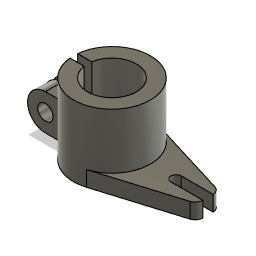
7.2 Project surface tools (Autodesk Fusion 360 design; units mm, degrees)
Autodesk Fusion 360 part; units mm, degrees
note: some values were not read from the file. Chosen so that the rebuilt part matches the saved one: which bodies a step acts on.
sketch "Sketch1" plane through (0, 0, 0) normal (0, 1, 0) x (1, 0, 0)
  circle A0 centre (0, 0) radius 19
  circle A1 centre (0, 0) radius 30
  line L0 (0, 0) -> (50, 0) construction
  line L1 (50, 0) -> (75, 0) construction
  line L2 (50, 4) -> (75, 4)
  line L3 (50, -4) -> (75, -4)
  line L4 (8.7717, 28.689) -> (70.7543, 9.7378)
  arc A2 (75, 4) -> (70.7543, 9.7378) centre (69, 4) ccw
  arc A3 (50, 4) -> (50, -4) centre (50, 0) ccw
  line L5 (8.7717, -28.689) -> (70.7543, -9.7378)
  arc A4 (70.7543, -9.7378) -> (75, -4) centre (69, -4) ccw
  dimension "d1" = 38
  dimension "d2" = 60
  dimension "d3" = 50
  dimension "d4" = 8
  dimension "d5" = 25
  dimension "d6" = 4
  dimension "d7" = 4
  dimension "d8" = 12
  constraint coincident A0.centre A1.centre
  constraint horizontal L0
  constraint coincident L0.end L1.start
  constraint parallel L0 L1
  constraint tangent A1 L4
  constraint coincident L2 A2.centre
  constraint tangent L4 A2
  constraint coincident A1 L4.start
  constraint symmetric L0 L2.end L3.end
  constraint symmetric L0 L4.end L5.end
  constraint symmetric L0 A2 A4
  constraint symmetric L0 L4.start L5.start
  measures "d1" diameter of A0
  measures "d2" diameter of A1
  measures "d3" distance of A0.centre L0.end
  measures "d4" diameter of A3
  measures "d5" distance of L0.end L1.end
  measures "d8" diameter of A2
extrude "Extrude1" add sketch "Sketch1" along normal blind 44 contours A1 makes body 1
extrude "Extrude2" add sketch "Sketch1" along normal blind 12 contours A1 L2 L3 L4 A2 A3 L5 A4 bodies 1
sketch "Sketch2" plane through (0, 0, 0) normal (0, 0, 1) x (1, 0, 0)
  circle A0 centre (-36, 22) radius 6
  line L0 (-36, 36) -> (-22, 36)
  line L1 (-22, 36) -> (-22, 8)
  line L2 (-22, 8) -> (-36, 8)
  arc A1 (-36, 36) -> (-36, 8) centre (-36, 22) ccw
  line L3 (30, 0) -> (-30, 0)
  dimension "d14" = 28
  dimension "d15" = 12
  dimension "d16" = 8
  dimension "d17" = 36
  constraint concentric A0 A1
  constraint horizontal L0
  constraint vertical L1
  constraint horizontal L2
  constraint tangent L2 A1
  constraint tangent L1 A1
  measures "d14" diameter of A1
  measures "d15" diameter of A0
  measures "d16" distance of L2 L3
  measures "d17" horizontal distance of origin A0.centre
extrude "Extrude3" add sketch "Sketch2" along normal mid plane 32 bodies 1
sketch "Sketch3" plane through (0, 44, 0) normal (0, 1, 0) x (-1, 0, 0)
  circle A0 centre (0, 0) radius 19
  circle A1 centre (0, 0) radius 30
  line L0 (54, -3) -> (11, -3)
  line L1 (11, -3) -> (11, 3)
  line L2 (11, 3) -> (54, 3)
  line L3 (54, 3) -> (54, -3)
  line L4 (0, 0) -> (-50, 0)
  dimension "d20" = 3
  dimension "d21" = 3
  dimension "d22" = 11
  dimension "d23" = 43
  constraint horizontal L0
  constraint vertical L1
  constraint horizontal L2
  constraint vertical L3
  measures "d20" distance of L0 L4
  measures "d21" distance of L2 L4
  measures "d22" distance of A0.centre L1
  measures "d23" distance of L1 L3
extrude "Extrude4" cut sketch "Sketch3" against normal up to surface (44 mm away) contours A0 A1 L0 L2 | A1 L0 L2 L3 bodies 1
extrude "Extrude5" add 1 faces at (26.2783, 44, 0) along direction (0, 1, 0) blind 11.305 on bodies 1 bodies 1
ref_plane "WorkPlane1" through (41.8858, 85.34, 0) normal (0, 1, 0) x (1, 0, 0)
ref_plane "WorkPlane2" through (0, 0, 57.35) normal (0, 0, 1) x (1, 0, 0)
sketch "Circle-project" plane through (41.8858, 85.34, 0) normal (0, 1, 0) x (1, 0, 0)
  circle A0 centre (-86.1816, 9.6942) radius 3.1596
sketch "sketch" plane through (0, 0, 57.35) normal (0, 0, 1) x (1, 0, 0)
  line L0 (-7.7739, 27.727) -> (8.0415, 27.727) construction
  line L1 (8.0415, 27.727) -> (8.0415, 37.727) construction
  line L2 (8.0415, 37.727) -> (-7.7739, 37.727) construction
  line L3 (-7.7739, 37.727) -> (-7.7739, 27.727) construction
  text T0 "360" font "Arial" height 10 bold align ink ink in box 0 x 0 at (-7.7639, 27.747) x (1, 0) y (0, 1) spacing 1 height is em
  constraint perpendicular L0 L1
  constraint parallel L0 L2
  constraint parallel L1 L3
extrude "Extrude6" add sketch "sketch" along normal blind 2.81 separate body text T0 makes body 2 at (7.5583, 30.8911, 57.35) makes body 3 at (-1.1306, 31.3924, 57.35) makes body 4 at (-4.9257, 31.7247, 57.35)
sketch "text" plane through (0, 0, 57.35) normal (0, 0, 1) x (1, 0, 0)
  line L0 (-7.7639, 29.7685) -> (-6.4358, 29.9296)
  spline S0 degree 3 poles (-6.4358, 29.9296) (-6.4097, 29.7744) (-6.3611, 29.4858) (-6.1784, 29.2583) (-6.094, 29.1532) knots 0 0 0 0 0.046307 0.086091 0.086091 0.086091 0.086091
  spline S1 degree 3 poles (-6.094, 29.1532) (-5.9959, 29.0749) (-5.7986, 28.9173) (-5.5468, 28.8956) (-5.4202, 28.8847) knots 0 0 0 0 0.036769 0.074001 0.074001 0.074001 0.074001
  spline S2 degree 3 poles (-5.4202, 28.8847) (-5.2839, 28.8984) (-5.0096, 28.9261) (-4.8068, 29.1129) (-4.7048, 29.2069) knots 0 0 0 0 0.039944 0.080374 0.080374 0.080374 0.080374
  spline S3 degree 3 poles (-4.7048, 29.2069) (-4.6202, 29.3289) (-4.4394, 29.5894) (-4.423, 29.9071) (-4.4143, 30.0761) knots 0 0 0 0 0.043667 0.093274 0.093274 0.093274 0.093274
  spline S4 degree 3 poles (-4.4143, 30.0761) (-4.4227, 30.2359) (-4.4384, 30.5366) (-4.6115, 30.7816) (-4.6926, 30.8964) knots 0 0 0 0 0.046906 0.088213 0.088213 0.088213 0.088213
  spline S5 degree 3 poles (-4.6926, 30.8964) (-4.79, 30.9847) (-4.9832, 31.16) (-5.2426, 31.1861) (-5.3713, 31.1991) knots 0 0 0 0 0.038332 0.076086 0.076086 0.076086 0.076086
  spline S6 degree 3 poles (-5.3713, 31.1991) (-5.4682, 31.1935) (-5.6816, 31.1811) (-5.8883, 31.1264) (-6.0012, 31.0966) knots 0 0 0 0 0.029044 0.063959 0.063959 0.063959 0.063959
  line L1 (-6.0012, 31.0966) -> (-5.8498, 32.2148)
  spline S7 degree 3 poles (-5.8498, 32.2148) (-5.6813, 32.2163) (-5.3745, 32.2191) (-5.1165, 32.3827) (-5.0002, 32.4565) knots 0 0 0 0 0.049359 0.089901 0.089901 0.089901 0.089901
  spline S8 degree 3 poles (-5.0002, 32.4565) (-4.9148, 32.5506) (-4.7395, 32.7438) (-4.7182, 33.0042) (-4.7073, 33.1376) knots 0 0 0 0 0.037062 0.076026 0.076026 0.076026 0.076026
  spline S9 degree 3 poles (-4.7073, 33.1376) (-4.7143, 33.25) (-4.7279, 33.4644) (-4.8595, 33.6334) (-4.9221, 33.7138) knots 0 0 0 0 0.032912 0.062778 0.062778 0.062778 0.062778
  spline S10 degree 3 poles (-4.9221, 33.7138) (-5.0021, 33.7764) (-5.1695, 33.9075) (-5.3823, 33.9214) (-5.4934, 33.9286) knots 0 0 0 0 0.029763 0.062314 0.062314 0.062314 0.062314
  spline S11 degree 3 poles (-5.4934, 33.9286) (-5.6062, 33.9185) (-5.8314, 33.8984) (-6.0066, 33.7557) (-6.094, 33.6845) knots 0 0 0 0 0.033159 0.066169 0.066169 0.066169 0.066169
  spline S12 degree 3 poles (-6.094, 33.6845) (-6.1694, 33.5882) (-6.3336, 33.3785) (-6.3746, 33.1144) (-6.3967, 32.9716) knots 0 0 0 0 0.036091 0.078606 0.078606 0.078606 0.078606
  line L2 (-6.3967, 32.9716) -> (-7.6614, 33.1864)
  spline S13 degree 3 poles (-7.6614, 33.1864) (-7.6163, 33.3851) (-7.5335, 33.7506) (-7.3481, 34.0757) (-7.2634, 34.224) knots 0 0 0 0 0.060707 0.111671 0.111671 0.111671 0.111671
  spline S14 degree 3 poles (-7.2634, 34.224) (-7.1638, 34.3475) (-6.9586, 34.6018) (-6.6698, 34.7554) (-6.5212, 34.8344) knots 0 0 0 0 0.047084 0.096979 0.096979 0.096979 0.096979
  spline S15 degree 3 poles (-6.5212, 34.8344) (-6.3549, 34.8992) (-6.0119, 35.0328) (-5.6439, 35.0485) (-5.4543, 35.0566) knots 0 0 0 0 0.053155 0.109642 0.109642 0.109642 0.109642
  spline S16 degree 3 poles (-5.4543, 35.0566) (-5.1382, 35.0339) (-4.5282, 34.9901) (-4.0592, 34.5999) (-3.8332, 34.412) knots 0 0 0 0 0.092479 0.17841 0.17841 0.17841 0.17841
  spline S17 degree 3 poles (-3.8332, 34.412) (-3.6866, 34.2336) (-3.4007, 33.8856) (-3.3534, 33.4384) (-3.3303, 33.2206) knots 0 0 0 0 0.067645 0.131876 0.131876 0.131876 0.131876
  spline S18 degree 3 poles (-3.3303, 33.2206) (-3.3838, 32.917) (-3.4984, 32.2655) (-4.0605, 31.9077) (-4.3606, 31.7167) knots 0 0 0 0 0.088546 0.189955 0.189955 0.189955 0.189955
  spline S19 degree 3 poles (-4.3606, 31.7167) (-4.1669, 31.6606) (-3.7866, 31.5503) (-3.5117, 31.2656) (-3.3767, 31.1259) knots 0 0 0 0 0.059338 0.116559 0.116559 0.116559 0.116559
  spline S20 degree 3 poles (-3.3767, 31.1259) (-3.2692, 30.9622) (-3.0483, 30.6259) (-3.0217, 30.2239) (-3.008, 30.0175) knots 0 0 0 0 0.057713 0.118596 0.118596 0.118596 0.118596
  spline S21 degree 3 poles (-3.008, 30.0175) (-3.0372, 29.7145) (-3.0958, 29.1059) (-3.4957, 28.6433) (-3.6965, 28.411) knots 0 0 0 0 0.088961 0.178675 0.178675 0.178675 0.178675
  spline S22 degree 3 poles (-3.6965, 28.411) (-3.9433, 28.2174) (-4.4465, 27.8224) (-5.085, 27.7724) (-5.4104, 27.747) knots 0 0 0 0 0.091931 0.1875 0.1875 0.1875 0.1875
  spline S23 degree 3 poles (-5.4104, 27.747) (-5.7162, 27.7666) (-6.3059, 27.8045) (-6.7891, 28.1431) (-7.0217, 28.3061) knots 0 0 0 0 0.08996 0.173509 0.173509 0.173509 0.173509
  spline S24 degree 3 poles (-7.0217, 28.3061) (-7.2129, 28.5095) (-7.6024, 28.9242) (-7.7094, 29.4835) (-7.7639, 29.7685) knots 0 0 0 0 0.081952 0.16704 0.16704 0.16704 0.16704
  spline S25 degree 3 poles (-0.6155, 30.2812) (-0.6081, 30.0778) (-0.5946, 29.7055) (-0.3974, 29.3911) (-0.3079, 29.2484) knots 0 0 0 0 0.059762 0.109449 0.109449 0.109449 0.109449
  spline S26 degree 3 poles (-0.3079, 29.2484) (-0.2056, 29.1424) (-0.0113, 28.9412) (0.2647, 28.9028) (0.3953, 28.8847) knots 0 0 0 0 0.042786 0.081231 0.081231 0.081231 0.081231
  spline S27 degree 3 poles (0.3953, 28.8847) (0.5173, 28.8975) (0.7632, 28.9233) (0.9406, 29.0957) (1.03, 29.1825) knots 0 0 0 0 0.035697 0.07196 0.07196 0.07196 0.07196
  spline S28 degree 3 poles (1.03, 29.1825) (1.1037, 29.3106) (1.2763, 29.6109) (1.2812, 29.9593) (1.2839, 30.1591) knots 0 0 0 0 0.043677 0.10237 0.10237 0.10237 0.10237
  spline S29 degree 3 poles (1.2839, 30.1591) (1.28, 30.3662) (1.2731, 30.7318) (1.0899, 31.0459) (1.0105, 31.182) knots 0 0 0 0 0.060871 0.107439 0.107439 0.107439 0.107439
  spline S30 degree 3 poles (1.0105, 31.182) (0.9144, 31.2767) (0.7239, 31.4643) (0.4584, 31.4927) (0.3269, 31.5067) knots 0 0 0 0 0.039235 0.077699 0.077699 0.077699 0.077699
  spline S31 degree 3 poles (0.3269, 31.5067) (0.1996, 31.4932) (-0.0583, 31.4657) (-0.2467, 31.2871) (-0.342, 31.1967) knots 0 0 0 0 0.037313 0.075584 0.075584 0.075584 0.075584
  spline S32 degree 3 poles (-0.342, 31.1967) (-0.4216, 31.0723) (-0.599, 30.7947) (-0.6096, 30.4638) (-0.6155, 30.2812) knots 0 0 0 0 0.043525 0.097125 0.097125 0.097125 0.097125
  line L3 (2.4949, 33.2743) -> (1.1668, 33.1278)
  spline S33 degree 3 poles (1.1668, 33.1278) (1.1481, 33.2513) (1.1142, 33.4755) (0.9753, 33.6534) (0.9128, 33.7333) knots 0 0 0 0 0.036712 0.066641 0.066641 0.066641 0.066641
  spline S34 degree 3 poles (0.9128, 33.7333) (0.8374, 33.7902) (0.6801, 33.9089) (0.4831, 33.9219) (0.3806, 33.9286) knots 0 0 0 0 0.027742 0.057804 0.057804 0.057804 0.057804
  spline S35 degree 3 poles (0.3806, 33.9286) (0.2397, 33.9101) (-0.053, 33.8716) (-0.2514, 33.6519) (-0.3542, 33.538) knots 0 0 0 0 0.041272 0.08569 0.08569 0.08569 0.08569
  spline S36 degree 3 poles (-0.3542, 33.538) (-0.4462, 33.3401) (-0.6842, 32.8277) (-0.7142, 32.2603) (-0.7327, 31.912) knots 0 0 0 0 0.064967 0.168253 0.168253 0.168253 0.168253
  spline S37 degree 3 poles (-0.7327, 31.912) (-0.5529, 32.0886) (-0.1976, 32.4377) (0.2972, 32.4911) (0.5418, 32.5175) knots 0 0 0 0 0.073265 0.14483 0.14483 0.14483 0.14483
  spline S38 degree 3 poles (0.5418, 32.5175) (0.8191, 32.4889) (1.3806, 32.4312) (1.8011, 32.054) (2.0139, 31.8632) knots 0 0 0 0 0.081433 0.16484 0.16484 0.16484 0.16484
  spline S39 degree 3 poles (2.0139, 31.8632) (2.1926, 31.6228) (2.5647, 31.1221) (2.6055, 30.4982) (2.6267, 30.1737) knots 0 0 0 0 0.08792 0.183155 0.183155 0.183155 0.183155
  spline S40 degree 3 poles (2.6267, 30.1737) (2.6054, 29.8315) (2.5647, 29.1784) (2.1701, 28.6585) (1.9822, 28.411) knots 0 0 0 0 0.100302 0.191447 0.191447 0.191447 0.191447
  spline S41 degree 3 poles (1.9822, 28.411) (1.7481, 28.2174) (1.2679, 27.8202) (0.6457, 27.7718) (0.3269, 27.747) knots 0 0 0 0 0.088875 0.182281 0.182281 0.182281 0.182281
  spline S42 degree 3 poles (0.3269, 27.747) (-0.0187, 27.7825) (-0.7116, 27.8536) (-1.207, 28.3436) (-1.4553, 28.5893) knots 0 0 0 0 0.100975 0.202492 0.202492 0.202492 0.202492
  spline S43 degree 3 poles (-1.4553, 28.5893) (-1.6578, 28.9519) (-2.1338, 29.8043) (-2.1464, 30.7863) (-2.1536, 31.3505) knots 0 0 0 0 0.122864 0.288763 0.288763 0.288763 0.288763
  spline S44 degree 3 poles (-2.1536, 31.3505) (-2.1456, 31.9298) (-2.1317, 32.9402) (-1.6371, 33.8144) (-1.426, 34.1874) knots 0 0 0 0 0.170286 0.297014 0.297014 0.297014 0.297014
  spline S45 degree 3 poles (-1.426, 34.1874) (-1.164, 34.4409) (-0.6362, 34.9516) (0.0953, 35.0214) (0.4636, 35.0566) knots 0 0 0 0 0.106024 0.213588 0.213588 0.213588 0.213588
  spline S46 degree 3 poles (0.4636, 35.0566) (0.7198, 35.0408) (1.2121, 35.0106) (1.6187, 34.7331) (1.8137, 34.6) knots 0 0 0 0 0.075393 0.144898 0.144898 0.144898 0.144898
  spline S47 degree 3 poles (1.8137, 34.6) (1.977, 34.4226) (2.325, 34.0446) (2.436, 33.5414) (2.4949, 33.2743) knots 0 0 0 0 0.071047 0.151424 0.151424 0.151424 0.151424
  spline S48 degree 3 poles (5.7273, 33.9189) (5.6464, 33.9122) (5.4842, 33.8988) (5.3502, 33.8064) (5.283, 33.7602) knots 0 0 0 0 0.023891 0.04792 0.04792 0.04792 0.04792
  spline S49 degree 3 poles (5.283, 33.7602) (5.2198, 33.6893) (5.0734, 33.5252) (5.014, 33.3123) (4.9802, 33.1913) knots 0 0 0 0 0.028131 0.065192 0.065192 0.065192 0.065192
  spline S50 degree 3 poles (4.9802, 33.1913) (4.9393, 32.9538) (4.8373, 32.3614) (4.8381, 31.7597) (4.8386, 31.3993) knots 0 0 0 0 0.072197 0.180043 0.180043 0.180043 0.180043
  spline S51 degree 3 poles (4.8386, 31.3993) (4.8372, 31.0441) (4.8348, 30.4633) (4.929, 29.8907) (4.9656, 29.6684) knots 0 0 0 0 0.10631 0.173818 0.173818 0.173818 0.173818
  spline S52 degree 3 poles (4.9656, 29.6684) (5.0029, 29.5318) (5.0664, 29.2993) (5.2214, 29.1164) (5.2854, 29.0409) knots 0 0 0 0 0.041785 0.071167 0.071167 0.071167 0.071167
  spline S53 degree 3 poles (5.2854, 29.0409) (5.3521, 28.9954) (5.4855, 28.9041) (5.6467, 28.8912) (5.7273, 28.8847) knots 0 0 0 0 0.023779 0.0476 0.0476 0.0476 0.0476
  spline S54 degree 3 poles (5.7273, 28.8847) (5.8082, 28.8914) (5.9704, 28.9048) (6.1044, 28.9971) (6.1716, 29.0434) knots 0 0 0 0 0.023891 0.04792 0.04792 0.04792 0.04792
  spline S55 degree 3 poles (6.1716, 29.0434) (6.2348, 29.1142) (6.3812, 29.2783) (6.4406, 29.4912) (6.4744, 29.6122) knots 0 0 0 0 0.028131 0.065192 0.065192 0.065192 0.065192
  spline S56 degree 3 poles (6.4744, 29.6122) (6.5153, 29.8485) (6.6175, 30.4392) (6.6166, 31.0393) (6.616, 31.3993) knots 0 0 0 0 0.071834 0.179559 0.179559 0.179559 0.179559
  spline S57 degree 3 poles (6.616, 31.3993) (6.6174, 31.7546) (6.6198, 32.3354) (6.5256, 32.9079) (6.489, 33.1303) knots 0 0 0 0 0.10631 0.173818 0.173818 0.173818 0.173818
  spline S58 degree 3 poles (6.489, 33.1303) (6.4516, 33.2669) (6.3878, 33.5) (6.2332, 33.684) (6.1692, 33.7602) knots 0 0 0 0 0.041842 0.071371 0.071371 0.071371 0.071371
  spline S59 degree 3 poles (6.1692, 33.7602) (6.1026, 33.8064) (5.9695, 33.8989) (5.808, 33.9122) (5.7273, 33.9189) knots 0 0 0 0 0.02387 0.047701 0.047701 0.047701 0.047701
  spline S60 degree 3 poles (5.7273, 35.0566) (6.0522, 35.0292) (6.6844, 34.976) (7.1345, 34.5308) (7.3533, 34.3144) knots 0 0 0 0 0.094491 0.183883 0.183883 0.183883 0.183883
  spline S61 degree 3 poles (7.3533, 34.3144) (7.5557, 33.9324) (8.0357, 33.0266) (8.0457, 31.9956) (8.0515, 31.3993) knots 0 0 0 0 0.128022 0.303575 0.303575 0.303575 0.303575
  spline S62 degree 3 poles (8.0515, 31.3993) (8.0451, 30.8035) (8.034, 29.7705) (7.5523, 28.8633) (7.3484, 28.4794) knots 0 0 0 0 0.175443 0.304172 0.304172 0.304172 0.304172
  spline S63 degree 3 poles (7.3484, 28.4794) (7.1305, 28.2658) (6.6808, 27.825) (6.0516, 27.7735) (5.7273, 27.747) knots 0 0 0 0 0.08865 0.182974 0.182974 0.182974 0.182974
  spline S64 degree 3 poles (5.7273, 27.747) (5.3964, 27.7798) (4.738, 27.845) (4.2737, 28.3159) (4.0427, 28.5502) knots 0 0 0 0 0.096473 0.191969 0.191969 0.191969 0.191969
  spline S65 degree 3 poles (4.0427, 28.5502) (3.8576, 28.9163) (3.4057, 29.8104) (3.4041, 30.8186) (3.4031, 31.414) knots 0 0 0 0 0.121617 0.296969 0.296969 0.296969 0.296969
  spline S66 degree 3 poles (3.4031, 31.414) (3.4097, 32.0073) (3.4212, 33.0371) (3.9023, 33.941) (4.1062, 34.3241) knots 0 0 0 0 0.174715 0.303221 0.303221 0.303221 0.303221
  spline S67 degree 3 poles (4.1062, 34.3241) (4.3241, 34.5377) (4.7738, 34.9785) (5.403, 35.03) (5.7273, 35.0566) knots 0 0 0 0 0.08865 0.182974 0.182974 0.182974 0.182974
delete_body "RemoveBody1" bodies 2
delete_body "RemoveBody2" bodies 4
delete_body "RemoveBody3" bodies 3
